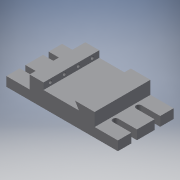
# Autodesk Inventor part: MVX-10-Bracket-V5
Saved by Autodesk Inventor 2016 (Build 200138000, 138)
## iProperties
Created: 2015-10-07
Part Number: MVX-10-Bracket-V5
Material: Generic
Document SubType Name: Modeling
Designer: voigt
Density: 1 g/cm^3
Appearance: Default
Author: voigt
Autodesk Inventor part; units mm, degrees
note: some values were not read from the file. Chosen so that the rebuilt part matches the saved one: direction of "Hole3".
ref_plane "YZ Plane" through (0, 0, 0) normal (1, 0, 0) x (0, 1, 0)
ref_plane "XZ Plane" through (0, 0, 0) normal (0, 1, 0) x (-1, 0, 0)
ref_plane "XY Plane" through (0, 0, 0) normal (0, 0, 1) x (1, 0, 0)
sketch "Sketch1" plane through (0, 0, 0) normal (0, 0, 1) x (1, 0, 0)
  line L0 (0, 57.1566) -> (0, -74.2716) construction
  line L1 (-84, 0) -> (84, 0) construction
  line L2 (-60, 30) -> (60, 30)
  line L3 (60, 30) -> (60, -30)
  line L4 (60, -30) -> (-60, -30)
  line L5 (-60, -30) -> (-60, 30)
  point P0 (0, 0)
  dimension "d0" = 120
  dimension "d1" = 60
  constraints: 8 end point, 2 parallel, 1 horizontal, 1 perpendicular, 2 other
  measures "d0" distance of L2.start L2.end
  measures "d1" distance of L2.end L3.end
extrude "Extrusion1" add sketch "Sketch1" along normal blind 24
sketch "Sketch2" plane through (-60, -30, 0) normal (0, -1, 0) x (1, 0, 0)
  line L0 (120, 24) -> (0, 24) projected
  line L1 (60, 28.8) -> (60, -4.8) construction
  line L2 (-24, 0) -> (144, 0) construction
  line L3 (41.9586, 17) -> (78.0414, 17) construction
  line L4 (41.9586, 17) -> (46.0001, 24) construction
  line L5 (41.9586, 17) -> (50.0416, 17) construction
  line L6 (78.0414, 17) -> (63.0829, 17) construction
  line L7 (73.9999, 24) -> (46.0001, 24) construction
  line L8 (73.9999, 24) -> (78.0414, 17)
  line L9 (78.0414, 17) -> (40, 17)
  line L10 (40, 17) -> (40, 24)
  line L11 (73.9999, 24) -> (40, 24)
  point P0 (60, 0)
  point P1 (77.464, 18)
  dimension "d5" = 60
  dimension "d7" = 7
  dimension "d37" = 1
  dimension "d39" = 17.464
  dimension "d40" = 60
  dimension "d64" = 20
  constraints: 18 end point, 5 point on line, 2 collinear, 2 horizontal, 1 equal length, 1 parallel, 1 perpendicular, 1 symmetric about line
  measures "d5" angle of L5 L4
  measures "d7" distance between parallel lines of L0 L3
  measures "d37" distance from line of L3 point (77.464, 18)
  measures "d39" distance from line of L1 point (77.464, 18)
  measures "d40" angle of L0 L8
  measures "d64" distance between parallel lines of L1 L10
extrude "Extrusion2" cut sketch "Sketch2" against normal up to next
sketch "Sketch9" plane through (0, 0, 24) normal (0, 0, 1) x (1, 0, 0)
  line L0 (0, 57.1566) -> (0, -74.2716) construction
  line L1 (-84, 0) -> (84, 0) construction
  line L2 (25, 37.3826) -> (25, -38.2478) construction
  line L3 (50, 36.5596) -> (50, -55.4961) construction
  line L4 (-25, 38.3811) -> (-25, -39.94) construction
  line L5 (-50, 35.8185) -> (-50, -44.962) construction
  line L6 (-20, -30) -> (-20, 30) construction
  line L7 (-60, 30) -> (-20, 30) construction
  line L8 (-60, -30) -> (-60, 30) construction
  line L9 (-20, -30) -> (-60, -30) construction
  line L10 (13.9999, 30) -> (13.9999, -30) construction
  line L11 (60, -30) -> (13.9999, -30) construction
  line L12 (60, 30) -> (60, -30) construction
  line L13 (13.9999, 30) -> (60, 30) construction
  line L14 (60, -30) -> (-60, -30) projected
  line L15 (-60, 30) -> (-35, 30)
  line L16 (-35, 30) -> (-35, -30)
  line L17 (-35, -30) -> (-60, -30)
  line L18 (-60, -30) -> (-60, 30)
  line L19 (13.9999, 30) -> (60, 30) projected
  line L20 (60, -30) -> (13.9999, -30) projected
  line L21 (60, 30) -> (35, 30)
  line L22 (35, 30) -> (35, -30)
  line L23 (35, -30) -> (60, -30)
  line L24 (60, -30) -> (60, 30)
  point P0 (0, 0)
  dimension "d65" = 25
  dimension "d66" = 25
  dimension "d67" = 25
  dimension "d68" = 25
  dimension "d69" = 25
  dimension "d70" = 25
  constraints: 24 end point, 4 parallel, 4 vertical, 2 horizontal, 2 perpendicular, 2 point on line
  measures "d65" distance between parallel lines of L0 L2
  measures "d66" distance between parallel lines of L2 L3
  measures "d67" distance between parallel lines of L0 L4
  measures "d68" distance between parallel lines of L4 L5
  measures "d69" distance of L16.end L17.end
  measures "d70" distance of L23.end L22.end
extrude "Extrusion7" cut sketch "Sketch9" against normal blind 14
sketch "Sketch10" plane through (0, 0, 10) normal (0, 0, 1) x (1, 0, 0)
  line L0 (-60, -30) -> (-60, 30) construction
  line L1 (-35, -30) -> (-60, -30) construction
  line L2 (-35, 30) -> (-35, -30) construction
  line L3 (-60, 30) -> (-35, 30) construction
  line L4 (60, -30) -> (35, -30) construction
  line L5 (60, 30) -> (60, -30) construction
  line L6 (35, 30) -> (60, 30) construction
  line L7 (35, -30) -> (35, 30) construction
  line L8 (-88.2, 0) -> (88.2, 0) construction
  line L9 (0, 42) -> (0, -42) construction
  line L10 (-60, -30) -> (-60, 30) construction
  line L11 (-60, 12.5) -> (60, 12.5) construction
  line L12 (60, 30) -> (60, -30) construction
  line L13 (-60, -12.5) -> (60, -12.5) construction
  line L14 (-60, 12.5) -> (-40, 12.5) construction
  line L15 (-60, 9.5) -> (-40, 9.5)
  line L16 (-40, 15.5) -> (-60, 15.5)
  arc A0 (-60, 15.5) -> (-60, 9.5) centre (-60, 12.5) ccw
  arc A1 (-40, 9.5) -> (-40, 15.5) centre (-40, 12.5) ccw
  line L17 (-60, -12.5) -> (-40, -12.5) construction
  line L18 (-60, -15.5) -> (-40, -15.5)
  line L19 (-40, -9.5) -> (-60, -9.5)
  arc A2 (-60, -9.5) -> (-60, -15.5) centre (-60, -12.5) ccw
  arc A3 (-40, -15.5) -> (-40, -9.5) centre (-40, -12.5) ccw
  line L20 (60, 12.5) -> (40, 12.5) construction
  line L21 (60, 15.5) -> (40, 15.5)
  line L22 (40, 9.5) -> (60, 9.5)
  arc A4 (60, 9.5) -> (60, 15.5) centre (60, 12.5) ccw
  arc A5 (40, 15.5) -> (40, 9.5) centre (40, 12.5) ccw
  line L23 (60, -12.5) -> (40, -12.5) construction
  line L24 (60, -9.5) -> (40, -9.5)
  line L25 (40, -15.5) -> (60, -15.5)
  arc A6 (60, -15.5) -> (60, -9.5) centre (60, -12.5) ccw
  arc A7 (40, -9.5) -> (40, -15.5) centre (40, -12.5) ccw
  point P0 (0, 0)
  point P1 (-50, 12.5)
  point P2 (-50, -12.5)
  point P3 (50, 12.5)
  point P4 (50, -12.5)
  dimension "d73" = 12.5
  dimension "d74" = 12.5
  dimension "d75" = 6
  dimension "d76" = 20
  dimension "d77" = 6
  dimension "d78" = 20
  dimension "d79" = 6
  dimension "d80" = 20
  dimension "d81" = 6
  dimension "d82" = 20
  constraints: 36 end point, 16 point on circle, 16 tangent, 8 centre point, 8 point on line, 4 midpoint, 4 parallel, 2 perpendicular
  measures "d73" distance between parallel lines of L8 L11
  measures "d74" distance between parallel lines of L13 L8
  measures "d75" diameter of A1
  measures "d76" distance from line of L0 L14.end
  measures "d77" diameter of A3
  measures "d78" distance of L11.end L20.end
  measures "d79" diameter of A5
  measures "d80" distance of L13.end L23.end
  measures "d81" diameter of A7
  measures "d82" distance from line of L0 L17.end
extrude "Extrusion8" cut sketch "Sketch10" against normal up to next
sketch "Sketch11" plane through (-35, -30, 24) normal (-1, 0, 0) x (0, 0, 1)
  line L0 (-7, 0) -> (-7, 60) construction
  line L1 (0, 60) -> (0, 0) construction
  line L2 (-14, 60) -> (0, 60) construction
  line L3 (-14, 60) -> (-14, 0) construction
  line L4 (0, 0) -> (-14, 0) construction
  line L5 (-3.5, 60) -> (-3.5, 0) construction
  line L6 (0, 0) -> (-14, 0) construction
  point P0 (-24, 30)
  point P1 (-3.5, 7.5)
  point P2 (-3.5, 22.5)
  point P3 (-3.5, 37.5)
  point P4 (-3.5, 52.5)
  dimension "d85" = 3.5
  dimension "d86" = 7.5
  dimension "d87" = 15
  dimension "d88" = 15
  dimension "d89" = 15
  constraints: 6 point on line, 2 end point, 1 vertical
  measures "d85" distance between parallel lines of L1 L5
  measures "d86" distance from line of L4 point (-3.5, 7.5)
  measures "d87" distance of point (-3.5, 22.5) point (-3.5, 7.5)
  measures "d88" distance of point (-3.5, 37.5) point (-3.5, 22.5)
  measures "d89" distance of point (-3.5, 52.5) point (-3.5, 37.5)
hole "Hole3" at (-35, -22.5, 20.5) at (-35, -7.5, 20.5) at (-35, 7.5, 20.5) at (-35, 22.5, 20.5) direction (1, 0, 0) diameter 3.242 end up to surface thread size "M4x0.7" class "6H" standard "ANSI Metric M Profile"
body "Solid1"
